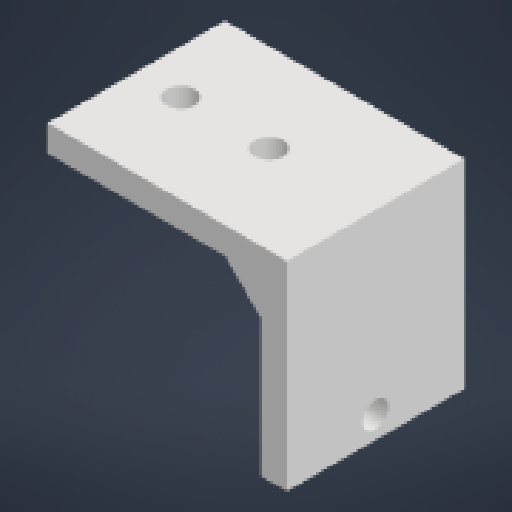
# Autodesk Inventor part: Motor_Holder
Saved by Autodesk Inventor 2026.1 (Build 301233020, 233B)
## iProperties
Created: 2025-10-16
Part Number: Motor_Holder
Material: Generic
Document SubType Name: Modeling
Designer: Garfieldcmix
Density: 1 g/cm^3
Appearance: Default
Author: Garfieldcmix
Autodesk Inventor part; units mm, degrees
ref_plane "YZ Plane" through (0, 0, 0) normal (1, 0, 0) x (0, 1, 0)
ref_plane "XZ Plane" through (0, 0, 0) normal (0, 1, 0) x (-1, 0, 0)
ref_plane "XY Plane" through (0, 0, 0) normal (0, 0, 1) x (1, 0, 0)
sketch "Sketch1" plane through (0, 0, 0) normal (0, 0, 1) x (1, 0, 0)
  line L0 (0, 22.5) -> (27, 22.5)
  line L1 (27, 22.5) -> (27, 0)
  line L2 (27, 0) -> (24, 0)
  line L3 (24, 0) -> (24, 19.5)
  line L4 (24, 19.5) -> (0, 19.5)
  line L5 (0, 19.5) -> (0, 22.5)
  line L6 (-5.4, 0) -> (32.4, 0) construction
  line L7 (0, -4.5) -> (0, 27) construction
  point P0 (0, 0)
  dimension "d0" = 3
  dimension "d1" = 3
  dimension "d2" = 22.5
  dimension "d3" = 27
  constraints: 12 end point, 4 perpendicular, 2 point on line, 1 horizontal, 1 parallel
  measures "d0" distance of L4.end L0.start
  measures "d1" distance of L1.end L2.end
  measures "d2" distance of L0.end L1.end
  measures "d3" distance of L0.start L0.end
extrude "Extrusion1" add sketch "Sketch1" along normal blind 20
chamfer "Chamfer1" distance 4 angle 45 1 edges at (24, 19.5, 10)
sketch "Sketch2" plane through (27, 0, 0) normal (1, 0, 0) x (0, 0, -1)
  circle A0 centre (-10, 2.5) radius 1.45
  line L0 (0, 0) -> (-20, 0) construction
  line L1 (-10, 0) -> (-10, 2.5) construction
  dimension "d9" = 2.9
  dimension "d10" = 2.5
  constraints: 2 end point, 1 centre point, 1 midpoint, 1 perpendicular
  measures "d9" diameter of A0
  measures "d10" distance of L1.start L1.end
extrude "Extrusion2" cut sketch "Sketch2" against normal up to surface (3 mm away)
sketch "Sketch3" plane through (0, 19.5, 0) normal (0, -1, 0) x (1, 0, 0)
  circle A0 centre (5, 10) radius 1.6
  circle A1 centre (15, 10) radius 1.6
  line L0 (0, 0) -> (0, 20) construction
  line L1 (0, 10) -> (20, 10) construction
  line L2 (20, 20) -> (20, 0) construction
  dimension "d13" = 3.2
  dimension "d14" = 5
  dimension "d15" = 5
  constraints: 2 centre point, 2 end point, 2 midpoint, 2 point on line, 1 equal radius
  measures "d13" diameter of A0
  measures "d14" distance from line of L0 A0.centre
  measures "d15" distance from line of L2 A1.centre
extrude "Extrusion3" cut sketch "Sketch3" against normal up to surface (3 mm away)
body "Solid1"
